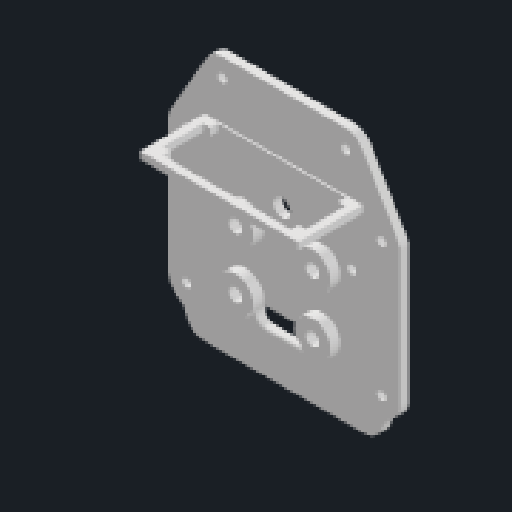
# Autodesk Inventor part: Sip_n_box
Saved by Autodesk Inventor 2024 (Build 280153000, 153)
## iProperties
Created: 2025-03-06
Part Number: Sip_n_box
Material: Generic
Document SubType Name: Modeling
Designer: colel
Density: 1 g/cm^3
Appearance: Default
Author: colel
Autodesk Inventor part; units mm, degrees
ref_plane "YZ Plane" through (0, 0, 0) normal (1, 0, 0) x (0, 1, 0)
ref_plane "XZ Plane" through (0, 0, 0) normal (0, 1, 0) x (-1, 0, 0)
ref_plane "XY Plane" through (0, 0, 0) normal (0, 0, 1) x (1, 0, 0)
sketch "Sketch1" plane through (0, 0, 0) normal (0, 0, 1) x (1, 0, 0)
  line L0 (-13.25, 10.25) -> (13.25, 10.25) construction
  line L1 (13.25, 10.25) -> (13.25, -10.25) construction
  line L2 (13.25, -10.25) -> (-13.25, -10.25) construction
  line L3 (-13.25, -10.25) -> (-13.25, 10.25) construction
  line L4 (-13.25, 10.25) -> (13.25, -10.25) construction
  line L5 (13.25, 10.25) -> (-13.25, -10.25) construction
  line L6 (25, 25) -> (-25, 25)
  line L7 (-25, 25) -> (-25, -25)
  line L8 (-25, -25) -> (25, -25)
  line L9 (25, -25) -> (25, 25)
  line L10 (25, 25) -> (-25, -25) construction
  line L11 (-25, 25) -> (25, -25) construction
  circle A0 centre (-13.25, 10.25) radius 2.25
  circle A1 centre (13.25, 10.25) radius 2.25
  circle A2 centre (13.25, -10.25) radius 2.25
  circle A3 centre (-13.25, -10.25) radius 2.25
  circle A4 centre (-13.25, 10.25) radius 6.25
  circle A5 centre (13.25, 10.25) radius 6.25
  circle A6 centre (13.25, -10.25) radius 6.25
  circle A7 centre (-13.25, -10.25) radius 6.25
  line L12 (-25, 25) -> (-25, 55)
  line L13 (-25, 55) -> (25, 55)
  line L14 (25, 55) -> (25, 25)
  point P0 (0, 0)
  dimension "d0" = 26.5
  dimension "d1" = 20.5
  dimension "d2" = 4.5
  dimension "d3" = 50
  dimension "d4" = 50
  dimension "d5" = 4
  dimension "d10" = 30
  constraints: 30 end point, 8 centre point, 6 equal radius, 4 coincident, 4 midpoint, 4 parallel, 4 perpendicular, 3 concentric, 2 horizontal, 1 vertical
  measures "d0" distance of L0.start L0.end
  measures "d1" distance of L2.end L0.start
  measures "d2" diameter of A0
  measures "d3" distance of L6.end L7.end
  measures "d4" distance of L6.start L6.end
  measures "d5" radial gap between concentric circles of A0 A4
  measures "d10" distance between parallel lines of L13 L6
extrude "Extrusion1" add sketch "Sketch1" against normal blind 3 contours L9 L8 L7 L6 | L6 L12 L13 L14 | A0 | A1 | A2 | A3 | A4 | A5 | A6 | A7
extrude "Extrusion2" add sketch "Sketch1" along normal blind 3.5 contours A4 | A5 | A6 | A7
sketch "Sketch2" plane through (0, 0, 0) normal (0, 0, 1) x (1, 0, 0)
  circle A0 centre (-13.25, 10.25) radius 6.25 projected
  circle A1 centre (13.25, 10.25) radius 6.25 projected
  line L0 (-25, 16.5) -> (25, 16.5) construction
  circle A2 centre (-13.25, 10.25) radius 6.25 projected
  circle A3 centre (13.25, -10.25) radius 6.25 projected
  circle A4 centre (-13.25, -10.25) radius 6.25 projected
  circle A5 centre (13.25, 10.25) radius 6.25 projected
  line L1 (-25, 55) -> (-25, -25) projected
  line L2 (-25, -25) -> (25, -25) projected
  line L3 (25, -25) -> (25, 55) projected
  line L4 (25, 55) -> (-25, 55) projected
  line L5 (-25, 26.5) -> (25, 26.5)
  line L6 (-25, 35) -> (25, 35)
  line L7 (-25, 32.5) -> (25, 32.5)
  point P0 (0, 0)
  dimension "d11" = 10
  dimension "d12" = 8.5
  dimension "d13" = 2.5
  constraints: 8 end point, 4 point on line, 2 parallel, 1 horizontal, 1 perpendicular, 1 tangent
  measures "d11" distance between parallel lines of L0 L5
  measures "d12" distance between parallel lines of L5 L6
  measures "d13" distance between parallel lines of L6 L7
extrude "Extrusion3" add sketch "Sketch2" along normal blind 20 contours L6 L3 L7 L1
sketch "Sketch4" plane through (0, 0, 0) normal (0, 0, 1) x (1, 0, 0)
  line L0 (-25, -25) -> (-25, 55) projected
  line L1 (-25, 55) -> (25, 55) projected
  line L2 (25, 55) -> (25, -25) projected
  line L3 (25, -25) -> (-25, -25) projected
  line L4 (-25, 55) -> (-40, 29.0192)
  line L5 (-40, 29.0192) -> (-40, -25)
  line L6 (-40, -25) -> (-25, -25)
  line L7 (25, -25) -> (40, -25)
  line L8 (40, -25) -> (40, 29.0192)
  line L9 (40, 29.0192) -> (25, 55)
  point P0 (0, 0)
  dimension "d27" = 15
  dimension "d28" = 15
  dimension "d29" = 30
  dimension "d30" = 30
  constraints: 12 end point, 2 perpendicular, 1 point on line, 1 vertical
  measures "d27" distance of L5.end L0.start
  measures "d28" distance of L2.end L7.end
  measures "d29" angle of L0 L4
  measures "d30" angle of L2 L9
extrude "Extrusion5" add sketch "Sketch4" against normal up to surface (3 mm away) contours L6 L5 L4 L0 | L2 L9 L8 L7
sketch "Sketch5" plane through (0, 0, 0) normal (0, 0, 1) x (1, 0, 0)
  arc A0 (1.0966, -13.3819) -> (-2.5966, -13.3819) centre (-0.75, 1) ccw projected
  circle A1 centre (-0.725, 20.1689) radius 3
  point P0 (0, 0)
  dimension "d33" = 6
  constraints: 1 centre point
  measures "d33" diameter of A1
extrude "Extrusion6" cut sketch "Sketch5" against normal through all
fillet "Fillet1" radius 6.35 6 edges at (-25, 55, -1.5) (25, 55, -1.5) (40, 29.0192, -1.5) (40, -25, -1.5) (-40, -25, -1.5) (-40, 29.0192, -1.5)
sketch "Sketch7" plane through (0, 0, 0) normal (0, 0, 1) x (1, 0, 0)
  arc A0 (-39.1493, 30.4928) -> (-40, 27.3178) centre (-33.65, 27.3178) ccw projected
  line L0 (-26.8331, 51.825) -> (-39.1493, 30.4928) projected
  arc A1 (-21.3338, 55) -> (-26.8331, 51.825) centre (-21.3338, 48.65) ccw projected
  line L1 (-21.3338, 55) -> (21.3338, 55) projected
  arc A2 (26.8331, 51.825) -> (21.3338, 55) centre (21.3338, 48.65) ccw projected
  line L2 (39.1493, 30.4928) -> (26.8331, 51.825) projected
  arc A3 (40, 27.3178) -> (39.1493, 30.4928) centre (33.65, 27.3178) ccw projected
  line L3 (40, -18.65) -> (40, 27.3178) projected
  arc A4 (33.65, -25) -> (40, -18.65) centre (33.65, -18.65) ccw projected
  line L4 (-33.65, -25) -> (33.65, -25) projected
  arc A5 (-40, -18.65) -> (-33.65, -25) centre (-33.65, -18.65) ccw projected
  line L5 (-40, 27.3178) -> (-40, -18.65) projected
  circle A6 centre (-0.725, 20.1689) radius 3 projected
  circle A7 centre (-21.3338, 48.65) radius 1.5
  circle A8 centre (21.3338, 48.65) radius 1.5
  circle A9 centre (33.65, 27.3178) radius 1.5
  circle A10 centre (-33.65, 27.3178) radius 1.5
  circle A11 centre (-33.65, -18.65) radius 1.5
  circle A12 centre (33.65, -18.65) radius 1.5
  point P0 (0, 0)
  dimension "d38" = 3
  dimension "d39" = 3
  dimension "d40" = 3
  dimension "d41" = 3
  dimension "d42" = 3
  dimension "d43" = 3
  constraints: 6 centre point
  measures "d38" diameter of A7
  measures "d39" diameter of A8
  measures "d40" diameter of A9
  measures "d41" diameter of A10
  measures "d42" diameter of A11
  measures "d43" diameter of A12
extrude "Extrusion7" cut sketch "Sketch7" against normal through all contours A7 | A8 | A9 | A10 | A11 | A12
sketch "Sketch8" plane through (0, 0, -3) normal (0, 0, -1) x (-1, 0, 0)
  circle A0 centre (-21.3338, 48.65) radius 1.5 projected
  circle A1 centre (33.65, -18.65) radius 1.5 projected
  circle A2 centre (33.65, 27.3178) radius 1.5 projected
  circle A3 centre (-33.65, 27.3178) radius 1.5 projected
  circle A4 centre (-33.65, -18.65) radius 1.5 projected
  circle A5 centre (21.3338, 48.65) radius 1.5 projected
  arc A6 (40, 27.3178) -> (39.1493, 30.4928) centre (33.65, 27.3178) ccw projected
  line L0 (26.8331, 51.825) -> (39.1493, 30.4928) projected
  arc A7 (26.8331, 51.825) -> (21.3338, 55) centre (21.3338, 48.65) ccw projected
  line L1 (21.3338, 55) -> (-21.3338, 55) projected
  arc A8 (-21.3338, 55) -> (-26.8331, 51.825) centre (-21.3338, 48.65) ccw projected
  line L2 (-39.1493, 30.4928) -> (-26.8331, 51.825) projected
  arc A9 (-39.1493, 30.4928) -> (-40, 27.3178) centre (-33.65, 27.3178) ccw projected
  line L3 (-40, -18.65) -> (-40, 27.3178) projected
  arc A10 (-40, -18.65) -> (-33.65, -25) centre (-33.65, -18.65) ccw projected
  line L4 (33.65, -25) -> (-33.65, -25) projected
  arc A11 (33.65, -25) -> (40, -18.65) centre (33.65, -18.65) ccw projected
  line L5 (40, 27.3178) -> (40, -18.65) projected
  circle A12 centre (0.725, 20.1689) radius 3 projected
  arc A13 (-36.5512, 28.9928) -> (-37, 27.3178) centre (-33.65, 27.3178) ccw construction
  line L6 (-36.5512, 28.9928) -> (-24.235, 50.325) construction
  arc A14 (-21.3338, 52) -> (-24.235, 50.325) centre (-21.3338, 48.65) ccw construction
  line L7 (-21.3338, 52) -> (21.3338, 52) construction
  arc A15 (24.235, 50.325) -> (21.3338, 52) centre (21.3338, 48.65) ccw construction
  line L8 (24.235, 50.325) -> (36.5512, 28.9928) construction
  arc A16 (37, 27.3178) -> (36.5512, 28.9928) centre (33.65, 27.3178) ccw construction
  line L9 (37, 27.3178) -> (37, -18.65) construction
  arc A17 (33.65, -22) -> (37, -18.65) centre (33.65, -18.65) ccw construction
  line L10 (33.65, -22) -> (-33.65, -22) construction
  arc A18 (-37, -18.65) -> (-33.65, -22) centre (-33.65, -18.65) ccw construction
  line L11 (-37, -18.65) -> (-37, 27.3178) construction
  line L12 (-6.35, -15.65) -> (6.35, -15.65) construction
  line L13 (-6.35, -18.825) -> (6.35, -18.825)
  line L14 (6.35, -12.475) -> (-6.35, -12.475)
  arc A19 (-6.35, -12.475) -> (-6.35, -18.825) centre (-6.35, -15.65) ccw
  arc A20 (6.35, -18.825) -> (6.35, -12.475) centre (6.35, -15.65) ccw
  point P0 (0, 0)
  point P1 (0, -15.65)
  dimension "d46" = 3
  dimension "d47" = 6.35
  dimension "d48" = 12.7
  dimension "d49" = 3.175
  constraints: 20 end point, 16 point on circle, 8 centre point, 4 tangent, 1 horizontal, 1 midpoint, 1 parallel, 1 vertical alignment, 11 other
  measures "d46" distance between parallel lines of L3 L11
  measures "d47" distance between parallel lines of L14 L13
  measures "d48" distance of L12.start L12.end
  measures "d49" distance between parallel lines of L13 L10
extrude "Extrusion8" cut sketch "Sketch8" against normal through all contours A19 L14 A20 L13
fillet "Fillet2" radius 0.7937 6 edges at (6.9326, -12.5289, 0) (-6.9326, -12.5289, 0) (0, -12.475, 0) (-8.7324, -17.7488, 0) (8.7324, -17.7488, 0) (0, -18.825, 0)
sketch "Sketch9" plane through (0, 0, -3) normal (0, 0, -1) x (-1, 0, 0)
  arc A0 (25.4131, 7.6083) -> (25.4131, 20.0295) centre (24.7125, 13.8189) ccw projected
  arc A1 (-23.9631, 20.0295) -> (-23.9631, 7.6083) centre (-23.2625, 13.8189) ccw projected
  circle A2 centre (-23.2625, 13.8189) radius 1.5
  circle A3 centre (24.7125, 13.8189) radius 1.5
  point P0 (0, 0)
  dimension "d53" = 3
  constraints: 2 centre point, 2 coincident, 1 equal radius
  measures "d53" diameter of A2
extrude "Extrusion9" cut sketch "Sketch9" against normal through all
sketch "Sketch10" plane through (0, 0, 0) normal (0, 0, 1) x (1, 0, 0)
  line L0 (-33.65, -25) -> (33.65, -25) projected
  line L1 (-33.65, -25) -> (-33.65, -33)
  line L2 (-33.65, -33) -> (33.65, -33)
  line L3 (33.65, -33) -> (33.65, -25)
  point P0 (0, 0)
  dimension "d56" = 8
  constraints: 6 end point, 2 perpendicular, 1 vertical
  measures "d56" distance of L0.start L1.end
extrude "Extrusion10" add sketch "Sketch10" against normal up to surface (3 mm away)
fillet "Fillet3" radius 6.35 4 edges at (-33.65, -25, -1.5) (33.65, -25, -1.5) (33.65, -33, -1.5) (-33.65, -33, -1.5)
sketch "Sketch12" plane through (-25, 35, 0) normal (0, 1, 0) x (1, 0, 0)
  line L0 (0.8174, -1.1484) -> (0.8174, -19.1484) projected
  line L1 (0.8174, -19.1484) -> (49.0174, -19.1484) projected
  line L2 (49.0174, -19.1484) -> (49.0174, -1.1484) projected
  line L3 (49.0174, -1.1484) -> (0.8174, -1.1484) projected
  line L4 (0, 0) -> (50, 0) projected
  line L5 (0, 0) -> (0, -20) projected
  line L6 (50, -20) -> (0, -20) projected
  line L7 (50, 0) -> (50, -20) projected
  line L8 (0, 0) -> (-2.3576, 0)
  line L9 (-2.3576, 0) -> (-2.3576, -22.3234)
  line L10 (-2.3576, -22.3234) -> (52.1924, -22.3234)
  line L11 (52.1924, -22.3234) -> (52.1924, 0)
  line L12 (52.1924, 0) -> (50, 0)
  point P0 (25, 0)
  dimension "d64" = 3.175
  dimension "d65" = 3.175
  dimension "d66" = 3.175
  constraints: 10 end point, 4 perpendicular, 1 horizontal, 1 point on line
  measures "d64" distance between parallel lines of L9 L0
  measures "d65" distance between parallel lines of L10 L1
  measures "d66" distance between parallel lines of L2 L11
extrude "Extrusion12" add sketch "Sketch12" against normal up to surface (2.5 mm away) contours L5 L6 L7 L12 L11 L10 L9 L8
sketch "Sketch13" plane through (-27.3576, 35, 22.3234) normal (0, 1, 0) x (1, 0, 0)
  line L0 (5.685, 3.785) -> (5.685, 5.325) construction
  line L1 (3.175, 3.175) -> (51.375, 3.175) construction
  line L2 (6.185, 5.825) -> (7.725, 5.825) construction
  line L3 (5.685, 19.025) -> (5.685, 20.565) construction
  line L4 (7.725, 18.525) -> (6.185, 18.525) construction
  line L5 (51.375, 3.175) -> (51.375, 21.175) construction
  line L6 (48.865, 5.325) -> (48.865, 3.785) construction
  line L7 (46.825, 5.825) -> (48.365, 5.825) construction
  line L8 (48.365, 18.525) -> (46.825, 18.525) construction
  line L9 (48.865, 20.565) -> (48.865, 19.025) construction
  line L10 (5.685, 20.565) -> (5.685, 21.175) construction
  line L11 (5.685, 19.025) -> (5.685, 18.525) construction
  line L12 (48.365, 18.525) -> (48.865, 18.525) construction
  line L13 (48.865, 18.525) -> (48.865, 19.025) construction
  line L14 (48.865, 20.565) -> (48.865, 21.175) construction
  line L15 (5.685, 3.785) -> (5.685, 3.175) construction
  line L16 (5.685, 5.325) -> (5.685, 5.825) construction
  line L17 (5.685, 5.825) -> (6.185, 5.825) construction
  line L18 (7.725, 5.825) -> (46.825, 5.825) construction
  line L19 (48.365, 5.825) -> (48.865, 5.825) construction
  line L20 (48.865, 5.825) -> (48.865, 5.325) construction
  line L21 (48.865, 3.785) -> (48.865, 3.175) construction
  line L22 (3.175, 5.825) -> (5.685, 5.825) construction
  line L23 (48.865, 5.825) -> (51.375, 5.825) construction
  line L24 (48.865, 18.525) -> (51.375, 18.525) construction
  line L25 (5.685, 18.525) -> (3.175, 18.525) construction
  line L26 (3.175, 18.525) -> (5.685, 18.525)
  line L27 (5.685, 21.175) -> (5.685, 18.525)
  line L28 (5.685, 21.175) -> (48.865, 21.175)
  line L29 (48.865, 18.525) -> (51.375, 18.525)
  line L30 (48.865, 21.175) -> (48.865, 18.525)
  line L31 (51.375, 18.525) -> (51.375, 5.825)
  line L32 (48.865, 3.175) -> (48.865, 5.825)
  line L33 (48.865, 5.825) -> (51.375, 5.825)
  line L34 (48.865, 3.175) -> (5.685, 3.175)
  line L35 (5.685, 3.175) -> (5.685, 5.825)
  line L36 (5.685, 5.825) -> (3.175, 5.825)
  line L37 (3.175, 5.825) -> (3.175, 18.525)
  line L38 (2.675, 19.025) -> (5.185, 19.025)
  line L39 (5.185, 19.025) -> (5.185, 21.675)
  line L40 (5.185, 21.675) -> (49.365, 21.675)
  line L41 (49.365, 21.675) -> (49.365, 19.025)
  line L42 (49.365, 19.025) -> (51.875, 19.025)
  line L43 (51.875, 19.025) -> (51.875, 5.325)
  line L44 (51.875, 5.325) -> (49.365, 5.325)
  line L45 (49.365, 5.325) -> (49.365, 2.675)
  line L46 (49.365, 2.675) -> (5.185, 2.675)
  line L47 (5.185, 2.675) -> (5.185, 5.325)
  line L48 (5.185, 5.325) -> (2.675, 5.325)
  line L49 (2.675, 5.325) -> (2.675, 19.025)
  point P0 (27.3576, 22.3234)
  dimension "d69" = 0.5
  constraints: 80 end point, 9 perpendicular, 9 point on line, 8 collinear, 2 horizontal, 2 parallel, 1 vertical, 11 other
  measures "d69" distance between parallel lines of L37 L49
extrude "Extrusion13" cut sketch "Sketch13" against normal up to surface (2.5 mm away) contours L26 L27 L28 L30 L29 L31 L33 L32 L34 L35 L36 L37 | L38 L39 L40 L41 L42 L43 L44 L45 L46 L47 L48 L49
fillet "Fillet4" radius 3.175 2 edges at (-27.3576, 33.75, 22.3234) (27.1924, 33.75, 22.3234)
fillet "Fillet5" radius 1.5875 2 edges at (-27.3576, 33.75, 0) (27.1924, 33.75, 0)
body "Solid1"
